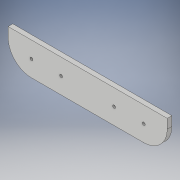
# Autodesk Inventor part: side drivetrain piece (8 wheel macanum)
Saved by Autodesk Inventor 2019 (Build 230136000, 136)
## iProperties
Created: 2019-04-20
Part Number: side drivetrain piece (8 wheel macanum)
Material: Generic
Document SubType Name: Modeling
Designer: Delta
Density: 1 g/cm^3
Appearance: Default
Author: Delta
Autodesk Inventor part; units mm, degrees
ref_plane "YZ Plane" through (0, 0, 0) normal (1, 0, 0) x (0, 1, 0)
ref_plane "XZ Plane" through (0, 0, 0) normal (0, 1, 0) x (-1, 0, 0)
ref_plane "XY Plane" through (0, 0, 0) normal (0, 0, 1) x (1, 0, 0)
sketch "Sketch1" plane through (0, 0, 0) normal (0, 0, 1) x (1, 0, 0)
  line L0 (-63.5, 0) -> (-368.3, 0)
  line L1 (-431.8, 63.5) -> (-431.8, 88.9)
  line L2 (-431.8, 88.9) -> (0, 88.9)
  line L3 (0, 88.9) -> (0, 63.5)
  arc A0 (-431.8, 63.5) -> (-368.3, 0) centre (-368.3, 63.5) ccw
  arc A1 (-63.5, 0) -> (0, 63.5) centre (-63.5, 63.5) ccw
  line L4 (-431.8, 88.9) -> (-287.8667, 88.9)
  line L5 (0, 88.9) -> (-143.9333, 88.9)
  point P0 (0, 0)
  point P1 (-431.8, 0)
  dimension "d0" = 431.8
  dimension "d1" = 88.9
  dimension "d2" = 63.5
  dimension "d3" = 63.5
  constraints: 12 end point, 4 point on circle, 4 point on line, 4 tangent, 3 horizontal, 2 centre point, 2 parallel, 1 perpendicular
  measures "d0" distance of L1.end L2.end
  measures "d1" distance of point (-431.8, 0) L1.end
  measures "d2" radius of A0
  measures "d3" radius of A1
extrude "Extrusion1" add sketch "Sketch1" along normal blind 12.7
sketch "Sketch2" plane through (0, 0, 12.7) normal (0, 0, 1) x (1, 0, 0)
  line L0 (-368.3, 0) -> (-63.5, 0) projected
  line L1 (0, 88.9) -> (-431.8, 88.9) projected
  line L2 (0, 63.5) -> (0, 88.9) projected
  line L3 (-431.8, 88.9) -> (-431.8, 63.5) projected
  point P0 (0, 0)
  point P1 (-368.3, 44.45)
  point P2 (-287.8667, 44.45)
  point P3 (-143.9333, 44.45)
  point P4 (-63.5, 44.45)
  dimension "d6" = 88.9
  dimension "d7" = 44.45
  dimension "d8" = 44.45
  dimension "d9" = 44.45
  dimension "d10" = 44.45
  dimension "d11" = 431.8
  dimension "d12" = 63.5
  dimension "d13" = 143.9333
  dimension "d14" = 143.9333
  dimension "d15" = 63.5
  measures "d6" distance between parallel lines of L0 L1
  measures "d7" distance from line of L1 point (-368.3, 44.45)
  measures "d8" distance from line of L1 point (-287.867, 44.45)
  measures "d9" distance from line of L1 point (-143.933, 44.45)
  measures "d10" distance from line of L1 point (-63.5, 44.45)
  measures "d11" distance between parallel lines of L2 L3
  measures "d12" distance from line of L3 point (-368.3, 44.45)
  measures "d13" distance from line of L3 point (-287.867, 44.45)
  measures "d14" distance from line of L2 point (-143.933, 44.45)
  measures "d15" distance from line of L2 point (-63.5, 44.45)
hole "Hole1" at (-368.3, 44.45, 12.7) at (-287.8667, 44.45, 12.7) at (-143.9333, 44.45, 12.7) at (-63.5, 44.45, 12.7) direction (0, 0, -1) diameter 7.9 end through all
equation "\"d7\" = 0.5 * d6"
equation "\"d8\" = 0.5 * d6"
equation "\"d9\" = 0.5 * d6"
equation "\"d10\" = 0.5 * d6"
equation "\"d13\" = 0.333333 * d11"
equation "\"d14\" = d13"
equation "\"d15\" = d12"
body "Solid1"
